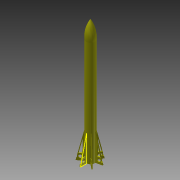
# Autodesk Inventor part: CTE Rocket
Saved by Autodesk Inventor 2014 (Build 180170000, 170)
## iProperties
Created: 2015-04-20
Part Number: CTE Rocket
Material: Generic
Document SubType Name: Modeling
Designer: stevehan
Density: 1 g/cm^3
Appearance: Yellow
Author: stevehan
Autodesk Inventor part; units mm, degrees
ref_plane "YZ Plane" through (0, 0, 0) normal (1, 0, 0) x (0, 1, 0)
ref_plane "XZ Plane" through (0, 0, 0) normal (0, 1, 0) x (-1, 0, 0)
ref_plane "XY Plane" through (0, 0, 0) normal (0, 0, 1) x (1, 0, 0)
sketch "Sketch1" plane through (0, 0, 0) normal (0, 1, 0) x (-1, 0, 0)
  circle A0 centre (0, 0) radius 12.7
  dimension "d0" = 25.4
  constraints: 1 centre point, 1 coincident
  measures "d0" diameter of A0
extrude "Extrusion1" add sketch "Sketch1" along normal blind 304.8
sketch "Sketch2" plane through (0, 0, 0) normal (1, 0, 0) x (0, 1, 0)
  line L0 (304.8, -12.7) -> (304.8, 12.7) projected
  line L1 (0, 12.7) -> (0, -12.7) projected
  line L2 (0, 12.7) -> (304.8, 12.7) projected
  line L3 (0, -12.7) -> (304.8, -12.7) projected
  line L4 (304.8, 0) -> (355.6, 0)
  line L5 (304.8, -12.7) -> (304.8, 0)
  arc A0 (304.8, -12.7) -> (355.6, 0) centre (310.799, 71.2542) ccw
  point P0 (0, 0)
  dimension "d3" = 50.8
  constraints: 4 end point, 2 point on circle, 1 centre point, 1 midpoint, 1 parallel, 1 perpendicular
  measures "d3" distance of L4.start L4.end
revolve "Revolution1" add sketch "Sketch2" angle 360 about axis through (0, 304.8, 0) along (0, 1, 0) contours L0 L4 A0
shell "Shell1" thickness 1.27 removed faces 1 at (3.6254, 0, -0.9542)
sketch "Sketch3" plane through (0, 0, 0) normal (0, -1, 0) x (1, 0, 0)
  circle A0 centre (0, 0) radius 11.43 projected
  line L0 (-1.27, 30.48) -> (1.27, 30.48)
  line L1 (1.27, 30.48) -> (1.27, 11.43)
  line L2 (1.27, 11.43) -> (-1.27, 11.43)
  line L3 (-1.27, 11.43) -> (-1.27, 30.48)
  dimension "d6" = 11.43
  dimension "d7" = 19.05
  dimension "d11" = 1.27
  dimension "d12" = 2.54
  constraints: 8 end point, 2 parallel, 1 horizontal, 1 perpendicular
  measures "d6" distance from line of A0.centre L2
  measures "d7" distance of L2.end L0.start
  measures "d11" distance from line of A0.centre L3
  measures "d12" distance of L0.start L0.end
extrude "Extrusion2" add sketch "Sketch3" against normal blind 76.2 contours L2 L3 L0 L1
sketch "Sketch4" plane through (1.27, 0, 30.48) normal (1, 0, 0) x (0, 0, -1)
  line L0 (0, 76.2) -> (17.8437, 76.2) projected
  line L1 (0, 0) -> (0, 76.2) projected
  line L2 (17.8437, 76.2) -> (0, 0)
  line L3 (0, 0) -> (-49.3647, 71.2935)
  line L4 (-49.3647, 71.2935) -> (-5.4781, 92.2343)
  line L5 (-5.4781, 92.2343) -> (17.8437, 76.2)
  point P0 (30.48, 0)
  constraints: 8 end point
extrude "Extrusion3" cut sketch "Sketch4" against normal blind 25.4 contours L0 L2 L1
sketch "Sketch5" plane through (1.27, 0, 30.48) normal (1, 0, 0) x (0, 0, -1)
  line L0 (17.8437, 76.2) -> (0, 0) projected
  line L1 (0, 0) -> (17.8437, 0) projected
  line L2 (17.8437, 76.2) -> (17.8437, 0) projected
  point P0 (30.48, 0)
sketch "Sketch6" plane through (-1.27, 0, 12.6363) normal (-1, 0, 0) x (0, 0, 1)
  line L0 (0, 0) -> (0, 76.2) projected
  circle A0 centre (7.9002, 9.9661) radius 4.4699
  line L1 (4.452, 12.9989) -> (4.452, 50.3362)
  line L2 (4.452, 50.3362) -> (8.9218, 16.1767)
  line L3 (8.9218, 16.1767) -> (4.452, 12.9989)
  point P0 (-12.6363, 0)
  constraints: 6 end point, 1 centre point, 1 parallel, 1 tangent
extrude "Extrusion4" cut sketch "Sketch6" against normal blind 25.4 contours A0
sketch "Sketch7" plane through (-1.27, 0, 12.6363) normal (-1, 0, 0) x (0, 0, 1)
  line L0 (17.8437, 0) -> (0, 76.2) projected
  line L1 (0, 0) -> (0, 76.2) projected
  line L2 (3.4304, 18.259) -> (3.4304, 53.7768)
  line L3 (3.4304, 53.7768) -> (11.7475, 18.259)
  line L4 (11.7475, 18.259) -> (3.4304, 18.259)
  point P0 (-12.6363, 0)
  constraints: 6 end point, 2 parallel, 1 perpendicular
extrude "Extrusion5" cut sketch "Sketch7" against normal blind 25.4
pattern_circular "Circular Pattern1" count 7 over 360 about axis through (0, 0, 0) along (0, 1, 0) of "Extrusion2", "Extrusion4", "Extrusion5", "Extrusion3"
body "Solid1"
